USB-C Cover (Autodesk Fusion 360 design; units mm, degrees)
Autodesk Fusion 360 part; units mm, degrees
sketch "Sketch1" plane through (0, 0, 0) normal (0, 0, 1) x (1, 0, 0)
  line L0 (0, 0) -> (-25, 0)
  line L1 (-25, 0) -> (-25, 28)
  line L2 (-25, 28) -> (0, 28)
  line L3 (0, 28) -> (0, 0)
  line L4 (-14.75, 25) -> (-10.25, 25)
  line L5 (-7.25, 22) -> (-7.25, 21.5)
  line L6 (-10.25, 18.5) -> (-14.75, 18.5)
  line L7 (-17.75, 21.5) -> (-17.75, 22)
  arc A0 (-10.25, 18.5) -> (-7.25, 21.5) centre (-10.25, 21.5) ccw
  arc A1 (-7.25, 22) -> (-10.25, 25) centre (-10.25, 22) ccw
  arc A2 (-14.75, 25) -> (-17.75, 22) centre (-14.75, 22) ccw
  arc A3 (-17.75, 21.5) -> (-14.75, 18.5) centre (-14.75, 21.5) ccw
  point P0 (-17.75, 25)
  point P1 (-17.75, 18.5)
  dimension "d1" = 25
  dimension "d2" = 28
  dimension "d3" = 6.5
  dimension "d4" = 10.5
  dimension "d5" = 3
  dimension "d6" = 7.25
  dimension "d9" = 3
  dimension "d10" = 3
  dimension "d11" = 3
  constraint horizontal L0
  constraint vertical L1
  constraint horizontal L2
  constraint vertical L3
  constraint coincident L0.start L3.end
  constraint horizontal L4
  constraint vertical L5
  constraint horizontal L6
  constraint vertical L7
  constraint tangent L5 A0
  constraint tangent L6 A0
  constraint tangent L4 A1
  constraint tangent L5 A1
  constraint coincident P0 L4
  constraint coincident P0 L7
  constraint tangent L4 A2
  constraint tangent L7 A2
  constraint equal A1 A2
  constraint coincident P1 L6
  constraint coincident P1 L7
  constraint tangent L6 A3
  constraint tangent L7 A3
  measures "d1" distance of L0.start L0.end
  measures "d2" distance of L0.start L2.end
  measures "d3" distance of P0 P1
  measures "d4" distance of L5 L7
  measures "d5" distance of L2 L4
  measures "d6" distance of L3 L5
  measures "d9" radius of A0
  measures "d10" radius of A1
  measures "d11" radius of A3
extrude "Extrude1" add sketch "Sketch1" along normal blind 1.2
